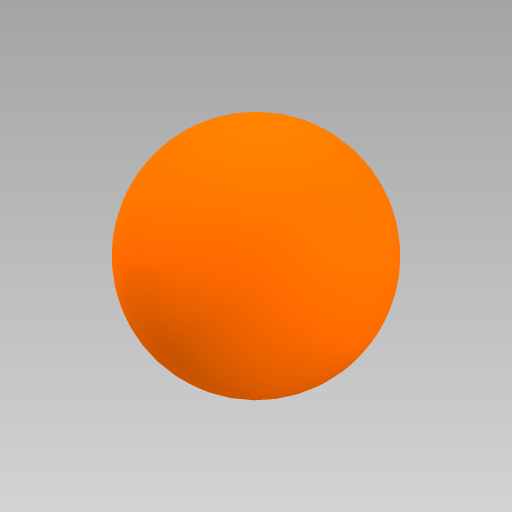
# Autodesk Inventor part: ball
Saved by Autodesk Inventor 2023.1 (Build 271208000, 208)
## iProperties
Created: 2023-12-16
Part Number: ball
Material: Типовые
Document SubType Name: Modeling
Designer: Фёдор
Density: 1 g/cm^3
Appearance: По умолчанию
Author: Фёдор
Autodesk Inventor part; units mm, degrees
ref_plane "YZ Plane" through (0, 0, 0) normal (1, 0, 0) x (0, 1, 0)
ref_plane "XZ Plane" through (0, 0, 0) normal (0, 1, 0) x (-1, 0, 0)
ref_plane "XY Plane" through (0, 0, 0) normal (0, 0, 1) x (1, 0, 0)
sketch "Эскиз1" plane through (0, 0, 0) normal (0, 1, 0) x (-1, 0, 0)
  arc A0 (21.5, 0) -> (-21.5, 0) centre (0, 0) ccw
  line L0 (-21.5, 0) -> (21.5, 0)
  arc A1 (-21.5, 0) -> (21.5, 0) centre (0, 0) ccw construction
  line L1 (21.5, 0) -> (64.1599, 0)
  dimension "d0" = 43
  constraints: 4 end point, 4 point on circle, 2 centre point, 2 horizontal, 1 coincident, 1 midpoint
  measures "d0" diameter of A0
revolve "Вращение1" add sketch "Эскиз1" angle 360 about axis through (-21.5, 0, 0) along (-1, 0, 0)
